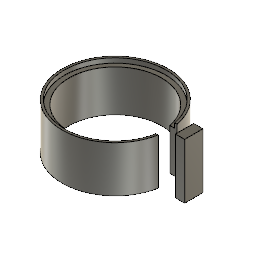
case v1 (Autodesk Fusion 360 design; units mm, degrees)
Autodesk Fusion 360 part; units mm, degrees
cylinder "CylinderPrimitive1" add diameter 115 height 50 placed x (1, 0, 0) y (0, 1, 0) z (0, 0, 1) at (0, 0, 0) makes body 1
hole "Hole1" at (0, 0, 50) direction (0, 0, -1) diameter 110 depth 5 tip angle 180 bodies 1
hole "Hole2" at (0, 0, 45) direction (0, 0, -1) diameter 100 end through all bodies 1
box "BoxPrimitive1" add length 20 width 10 height 60 placed x (0, 1, 0) y (-1, 0, 0) z (0, 0, 1) at (85, -10, 0) separate body makes body 2
extrude "Extrude1" cut 1 faces at (75, 3.3333, 20) along direction (-1, 0, 0) blind 40 on bodies 2 bodies 1
